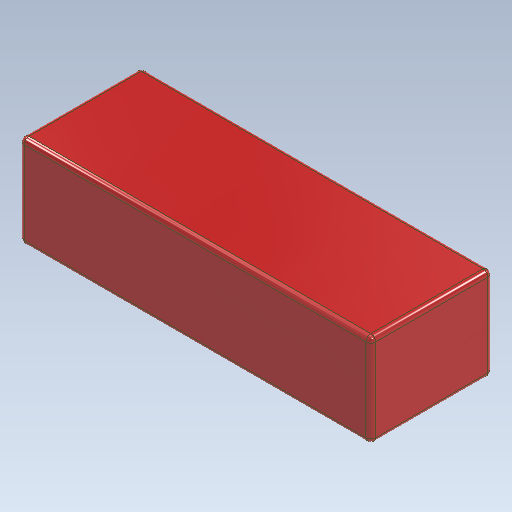
# Autodesk Inventor part: Battery[72x25x19]
Saved by Autodesk Inventor 2020 (Build 240168000, 168)
## iProperties
Created: 2019-12-14
Part Number: Battery[72x25x19]
Material: Polypropylene
Document SubType Name: Modeling
Designer: ermoz
Density: 0.899 g/cm^3
Appearance: Smooth - Ash
Mass: 30.6575 g
Surface Area: 70.8572 cm^2
Volume: 34.1018 cm^3
Author: ermoz
Autodesk Inventor part; units mm, degrees
ref_plane "YZ Plane" through (0, 0, 0) normal (1, 0, 0) x (0, 1, 0)
ref_plane "XZ Plane" through (0, 0, 0) normal (0, 1, 0) x (-1, 0, 0)
ref_plane "XY Plane" through (0, 0, 0) normal (0, 0, 1) x (1, 0, 0)
sketch "Sketch1" plane through (0, 0, 0) normal (0, 1, 0) x (-1, 0, 0)
  line L0 (0, 0) -> (72, 0)
  line L1 (72, 0) -> (72, -25)
  line L2 (72, -25) -> (0, -25)
  line L3 (0, -25) -> (0, 0)
  dimension "d0" = 72
  dimension "d1" = 25
  constraints: 8 end point, 2 parallel, 1 horizontal, 1 perpendicular
  measures "d0" distance of L1.end L2.end
  measures "d1" distance of L0.end L1.end
extrude "Extrusion1" add sketch "Sketch1" along normal blind 19
fillet "Fillet1" radius 1 3 edges at (-36, 19, 0) (0, 9.5, 0) (0, 19, -12.5)
fillet "Fillet2" radius 1 12 edges at (-0.2929, 0, -0.2929) (0, 0, -13) (-36.5, 0, 0) (-36, 0, -25) (-72, 0, -12.5) (-72, 18.7071, -0.2929) (-72, 19, -13) (-72, 9, 0) (-72, 9.5, -25) (-0.2929, 18.7071, -25) (0, 9, -25) (-36.5, 19, -25)
body "Solid1"
